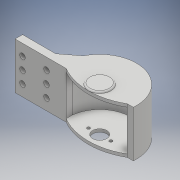
# Autodesk Inventor part: Omni Encoder-trackers
Saved by Autodesk Inventor 2018 (Build 220112000, 112)
## iProperties
Created: 2018-03-22
Part Number: Omni Encoder-trackers
Material: Generic
Document SubType Name: Modeling
Designer: Kelly
Density: 1 g/cm^3
Appearance: Default
Author: Kelly
Autodesk Inventor part; units mm, degrees
ref_plane "YZ Plane" through (0, 0, 0) normal (1, 0, 0) x (0, 1, 0)
ref_plane "XZ Plane" through (0, 0, 0) normal (0, 1, 0) x (-1, 0, 0)
sketch "Sketch1" plane through (0, 0, 0) normal (0, 0, 1) x (1, 0, 0)
  circle A0 centre (0, 0) radius 4.75
  circle A1 centre (0, 0) radius 17.5 construction
  arc A2 (20.4022, -2) -> (-20.4022, -2) centre (0, 0) ccw
  arc A3 (-20.4022, -2) -> (20.4022, -2) centre (0, 33.0909) ccw
  arc A4 (-20.4022, -2) -> (20.4022, -2) centre (0, 0) ccw construction
  arc A5 (24.4182, -2) -> (-24.4182, -2) centre (0, 0) ccw
  line L0 (-20.4022, -2) -> (-24.4182, -2)
  line L1 (20.4022, -2) -> (24.4182, -2)
  arc A6 (-24.4182, -2) -> (24.4182, -2) centre (0, 0) ccw construction
  dimension "d0" = 9.5
  dimension "d1" = 35
  dimension "d2" = 41
  dimension "d3" = 10
  dimension "d4" = 2
  dimension "d5" = 49
  constraints: 10 point on circle, 7 centre point, 4 coincident, 4 end point, 2 horizontal, 1 horizontal alignment
  measures "d0" diameter of A0
  measures "d1" diameter of A1
  measures "d2" diameter of A2
  measures "d4" vertical distance of L0.start point (0, 0)
  measures "d5" diameter of A5
extrude "Extrusion1" add sketch "Sketch1" along normal blind 2
extrude "Extrusion2" add sketch "Sketch1" against normal blind 13.5 contours A2 L0 A5 L1
mirror "Mirror1" about plane through (0, 12.5652, -13.5) normal (0, 0, -1) of "Extrusion1", "Extrusion2"
sketch "Sketch2" plane through (0, 0, -29) normal (0, 0, -1) x (-1, 0, 0)
  circle A0 centre (0, 0) radius 7.45
  circle A1 centre (7.45, 0) radius 1
  circle A2 centre (-7.45, 0) radius 1
  point P0 (0, 7.45)
  dimension "d10" = 14.9
  dimension "d11" = 2
  dimension "d14" = 360
  dimension "d16" = 90
  constraints: 3 centre point, 2 point on circle, 1 coincident, 1 vertical alignment, 5 other
  measures "d10" diameter of A0
  measures "d11" diameter of A1
extrude "Extrusion3" cut sketch "Sketch2" against normal up to surface (2 mm away) contours A0 A1 | A0 A1 | A2 A0 | A0 A2
sketch "Sketch3" plane through (0, 0, 2) normal (0, 0, 1) x (1, 0, 0)
  circle A0 centre (0, 0) radius 7.5
  dimension "d19" = 15
  constraints: 1 centre point, 1 coincident
  measures "d19" diameter of A0
extrude "Extrusion4" add sketch "Sketch3" along normal blind 1
fillet "Fillet1" radius 1 1 edges at (-7.5, 0, 3)
sketch "Sketch7" plane through (-24.4182, -2, 2) normal (0, -1, 0) x (1, 0, 0)
  line L0 (4.016, -2) -> (4.016, 0) projected
  line L1 (0, 0) -> (4.016, 0) projected
  line L2 (0, -31) -> (0, 0) projected
  line L3 (0, -31) -> (4.016, -31) projected
  line L4 (4.016, -29) -> (4.016, -31) projected
  line L5 (4.016, -2) -> (4.016, -29) projected
  line L6 (44.8204, -31) -> (4.016, -31) projected
  line L7 (4.016, -31) -> (-30, -31)
  line L8 (-30, -31) -> (-30, 0)
  line L9 (-30, 0) -> (4.016, 0)
  line L10 (4.016, 0) -> (4.016, -31)
  point P0 (24.4182, -2)
  dimension "d36" = 30
  constraints: 8 end point, 2 parallel, 1 horizontal, 1 perpendicular, 1 point on line
  measures "d36" distance between parallel lines of L8 L2
extrude "Extrusion8" add sketch "Sketch7" against normal blind 5
sketch "Sketch8" plane through (0, 33.0909, -29) normal (0, 0, -1) x (-1, 0, 0)
  arc A0 (24.3156, -30.0909) -> (-24.4182, -35.0909) centre (0, -33.0909) ccw projected
  line L0 (-20.4022, -35.0909) -> (-24.4182, -35.0909) projected
  arc A1 (-20.4022, -35.0909) -> (20.4022, -35.0909) centre (0, 0) ccw projected
  line L1 (54.4182, -35.0909) -> (20.4022, -35.0909) projected
  line L2 (54.4182, -35.0909) -> (54.4182, -30.0909) projected
  line L3 (24.3156, -30.0909) -> (54.4182, -30.0909) projected
  circle A2 centre (-7.45, -33.0909) radius 1 projected
  circle A3 centre (7.45, -33.0909) radius 1 projected
  circle A4 centre (0, -33.0909) radius 4.75 projected
  arc A5 (24.3156, -30.0909) -> (-24.4182, -35.0909) centre (0, -33.0909) ccw projected
  line L4 (21.8918, -22.0909) -> (32.3156, -30.0909)
  line L5 (54.4182, -30.0909) -> (24.3156, -30.0909) projected
  dimension "d39" = 8
  dimension "d40" = 8
  constraints: 2 end point, 1 point on circle, 1 point on line
  measures "d39" distance of L4.end L3.start
  measures "d40" vertical distance of L3.start L4.start
extrude "Extrusion9" add sketch "Sketch8" against normal blind 2 contours A0 L4 L3
ref_plane "Work Plane2" through (0, 0, -13.5) normal (0, 0, 1) x (1, 0, 0)
mirror "Mirror4" about plane through (0, 0, -13.5) normal (0, 0, 1) of "Extrusion9"
sketch "Sketch9" plane through (-24.4182, 3, 2) normal (0, 1, 0) x (1, 0, 0)
  line L0 (-7.8974, 0) -> (-7.8974, 2) projected
  line L1 (-7.8974, 2) -> (0.1026, 2) projected
  line L2 (0.1026, 29) -> (0.1026, 2) projected
  line L3 (0.1026, 29) -> (-7.8974, 29) projected
  line L4 (-7.8974, 29) -> (-7.8974, 31) projected
  line L5 (-7.8974, 31) -> (-30, 31) projected
  line L6 (-30, 31) -> (-30, 0) projected
  line L7 (-30, 0) -> (-7.8974, 0) projected
  point P0 (24.4182, 2)
  point P1 (-25, 7.5)
  point P2 (-25, 15.5)
  point P3 (-25, 23.5)
  point P4 (-9, 7.5)
  point P5 (-9, 15.5)
  point P6 (-9, 23.5)
  dimension "d45" = 8
  dimension "d48" = 16
  dimension "d51" = 31
  dimension "d52" = 7.5
  dimension "d53" = 5
  constraints: 1 horizontal, 1 vertical, 5 other
  measures "d45" distance of point (-25, 7.5) point (-25, 15.5)
  measures "d48" distance of point (-25, 7.5) point (-9, 7.5)
  measures "d51" distance of L5.end L6.end
  measures "d52" distance from line of L7 point (-25, 7.5)
  measures "d53" distance from line of L6 point (-25, 7.5)
hole "Hole1" at (-49.4182, 3, -5.5) at (-49.4182, 3, -13.5) at (-49.4182, 3, -21.5) at (-33.4182, 3, -5.5) at (-33.4182, 3, -13.5) at (-33.4182, 3, -21.5) direction (0, -1, 0) diameter 3.7 end through all
body "Solid1"
